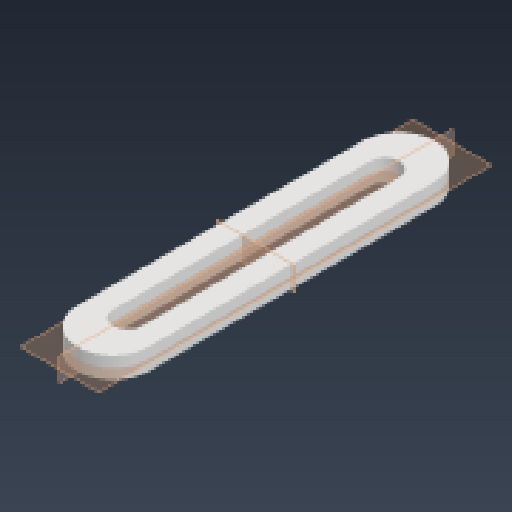
# Autodesk Inventor part: Качалка_крепления_камеры
Saved by Autodesk Inventor 2023.2 (Build 272271030, 271C)
## iProperties
Created: 2025-10-07
Part Number: Качалка_крепления_камеры
Material: Типовые
Document SubType Name: Modeling
Designer: Олег Коноваленко
Density: 1 g/cm^3
Appearance: По умолчанию
Author: Олег Коноваленко
Autodesk Inventor part; units mm, degrees
sketch "Эскиз1" plane through (0, 0, 0) normal (0, 1, 0) x (-1, 0, 0)
  line L0 (0, 35) -> (0, -35) construction
  line L1 (-5, 35) -> (-5, -35)
  line L2 (5, -35) -> (5, 35)
  arc A0 (5, 35) -> (-5, 35) centre (0, 35) ccw
  arc A1 (-5, -35) -> (5, -35) centre (0, -35) ccw
  line L3 (0, 23.8) -> (0, -13) construction
  line L4 (-1.6, 23.8) -> (-1.6, -13)
  line L5 (1.6, -13) -> (1.6, 23.8)
  arc A2 (1.6, 23.8) -> (-1.6, 23.8) centre (0, 23.8) ccw
  arc A3 (-1.6, -13) -> (1.6, -13) centre (0, -13) ccw
  line L6 (-7, 0) -> (7, 0) projected
  circle A4 centre (0, -35) radius 2.1
  point P0 (-5, 0)
  point P1 (-1.6, 0)
  point P2 (1.6, 0)
  point P3 (5, 0)
  point P4 (0, 0)
  point P5 (0, 25.4)
  point P6 (0, -14.6)
  dimension "d0" = 10
  dimension "d1" = 70
  dimension "d2" = 3.2
  dimension "d6" = 4.2
  dimension "d7" = 22
  dimension "d8" = 40
  constraints: 16 end point, 10 point on circle, 8 tangent, 5 centre point, 2 parallel, 2 point on line, 1 concentric, 1 midpoint, 1 vertical
  measures "d0" distance between parallel lines of L1 L2
  measures "d1" distance of L0.start L0.end
  measures "d2" distance between parallel lines of L4 L5
  measures "d6" diameter of A4
  measures "d7" distance of L3.end A4.centre
  measures "d8" distance of point (0, 25.4) point (0, -14.6)
extrude "Выдавливание1" add sketch "Эскиз1" along normal mid plane 3 contours A0 L2 L6 L5 A2 L4 L1 | L6 L4 A3 L5 L2 A1 L1
